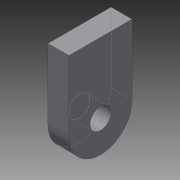
# Autodesk Inventor part: Battey latch
Saved by Autodesk Inventor 2015 (Build 190159000, 159)
## iProperties
Created: 2014-11-13
Part Number: Battey latch
Material: Generic
Document SubType Name: Modeling
Designer: karl
Density: 1 g/cm^3
Appearance: Default
Author: karl
Autodesk Inventor part; units mm, degrees
ref_plane "YZ Plane" through (0, 0, 0) normal (1, 0, 0) x (0, 1, 0)
ref_plane "XZ Plane" through (0, 0, 0) normal (0, 1, 0) x (-1, 0, 0)
ref_plane "XY Plane" through (0, 0, 0) normal (0, 0, 1) x (1, 0, 0)
sketch "Sketch1" plane through (0, 0, 0) normal (1, 0, 0) x (0, 1, 0)
  line L0 (-4.5, 7.5) -> (4.5, 7.5)
  line L1 (4.5, 7.5) -> (4.5, -7.5)
  line L2 (4.5, -7.5) -> (-4.5, -7.5)
  line L3 (-4.5, -7.5) -> (-4.5, 7.5)
  line L4 (-4.5, 7.5) -> (4.5, -7.5) construction
  line L5 (4.5, 7.5) -> (-4.5, -7.5) construction
  circle A0 centre (0, -7.5) radius 4.5
  point P0 (0, 0)
  dimension "d0" = 9
  dimension "d1" = 15
  dimension "d2" = 9
  constraints: 12 end point, 3 midpoint, 2 parallel, 1 centre point, 1 horizontal, 1 perpendicular
  measures "d0" distance of L1.end L2.end
  measures "d1" distance of L0.end L1.end
  measures "d2" diameter of A0
extrude "Extrusion1" add sketch "Sketch1" along normal blind 3
sketch "Sketch2" plane through (0, 0, 0) normal (-1, 0, 0) x (0, 0, 1)
  arc A0 (-7.5, 4.5) -> (-7.5, -4.5) centre (-7.5, 0) ccw projected
  circle A1 centre (-7.5, 0) radius 1.5
  point P0 (0, 0)
  dimension "d5" = 3
  constraints: 1 centre point, 1 coincident
  measures "d5" diameter of A1
extrude "Extrusion2" cut sketch "Sketch2" against normal blind 10
sketch "Sketch3" plane through (0, 0, 0) normal (-1, 0, 0) x (0, 0, 1)
  line L0 (7.5, -4.5) -> (-7.5, -4.5) projected
  line L1 (0.5, -4.5) -> (5.5, -4.5)
  line L2 (5.5, -4.5) -> (5.5, -7.5)
  line L3 (5.5, -7.5) -> (0.5, -7.5)
  line L4 (0.5, -7.5) -> (0.5, -4.5)
  circle A0 centre (-7.5, 0) radius 1.5 projected
  point P0 (0, 0)
  dimension "d8" = 5
  dimension "d9" = 3
  dimension "d10" = 8
  constraints: 8 end point, 2 parallel, 1 horizontal, 1 perpendicular, 1 point on line
  measures "d8" distance of L2.end L3.end
  measures "d9" distance of L1.end L2.end
  measures "d10" distance from line of L4 A0.centre
extrude "Extrusion3" add sketch "Sketch3" against normal blind 3 contours L2 L3 L4 L0
body "Solid1"
